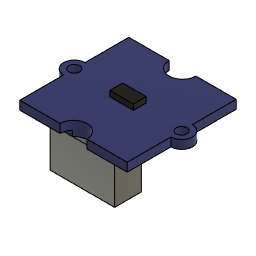
tofBreakoutBoard v3 (Autodesk Fusion 360 design; units mm, degrees)
Autodesk Fusion 360 part; units mm, degrees
sketch "Esquisse1" plane through (0, 0, 0) normal (0, 0, 1) x (1, 0, 0)
  line L0 (10, 13.25) -> (10, 7.05) construction
  line L1 (-3, 10.15) -> (23, 10.15) construction
  circle A0 centre (20, 10.15) radius 1
  circle A1 centre (0, 10.15) radius 1
  arc A2 (7.5, 20.3) -> (12.5, 20.3) centre (10, 20.3) ccw
  line L2 (20, 20.3) -> (12.5, 20.3)
  line L3 (7.5, 20.3) -> (0, 20.3)
  line L4 (20, 0) -> (20, 8.15)
  line L5 (20, 12.15) -> (20, 20.3)
  arc A3 (20, 8.15) -> (20, 12.15) centre (20, 10.15) ccw
  line L6 (0, 0) -> (7.5, 0)
  line L7 (12.5, 0) -> (20, 0)
  arc A4 (12.5, 0) -> (7.5, 0) centre (10, 0) ccw
  line L8 (0, 20.3) -> (0, 12.15)
  line L9 (0, 8.15) -> (0, 0)
  arc A5 (0, 12.15) -> (0, 8.15) centre (0, 10.15) ccw
  line L10 (0, 0) -> (20, 20.3) construction
  line L11 (0, 20.3) -> (20, 0) construction
  dimension "d1" = 20
  dimension "d2" = 20.3
  dimension "d3" = 5
  dimension "d4" = 5
  dimension "d5" = 4
  dimension "d6" = 4
  dimension "d7" = 2
  dimension "d8" = 2
  constraint horizontal L6
  constraint vertical L4
  constraint horizontal L2
  constraint vertical L8
  constraint coincident L6.start L9.end
  constraint parallel L0 L4
  constraint horizontal L1
  constraint concentric A0 A3
  constraint concentric A1 A5
  constraint coincident A2.start L2
  constraint collinear L2 L3
  constraint collinear L4 L5
  constraint coincident A0.centre L4
  constraint collinear L6 L7
  constraint coincident A4.centre L6
  constraint coincident A1.centre L8
  constraint midpoint L1 L10
  constraint midpoint L0 L1
  constraint coincident L0 A2.centre
  constraint coincident L0 A4.centre
  constraint coincident L1 A0.centre
  constraint coincident L1 A1.centre
  constraint collinear L8 L9
  constraint coincident A2.centre L2
  measures "d1" distance of L2.start L3.end
  measures "d2" distance of L4.start L2.start
  measures "d3" diameter of A4
  measures "d4" diameter of A2
  measures "d5" diameter of A3
  measures "d6" diameter of A5
  measures "d7" diameter of A1
  measures "d8" diameter of A0
extrude "Extrusion1" add sketch "Esquisse1" along normal blind 1.6 makes body 1
sketch "Esquisse2" plane through (0, 0, 1.6) normal (0, 0, 1) x (-1, 0, 0)
  circle A0 centre (-20, -10.15) radius 1
  circle A1 centre (0, -10.15) radius 1
  line L0 (-7.5, -20.3) -> (0, -20.3)
  line L1 (0, -20.3) -> (0, -12.15)
  arc A2 (0, -12.15) -> (0, -8.15) centre (0, -10.15) ccw
  line L2 (0, -8.15) -> (0, 0)
  line L3 (0, 0) -> (-7.5, 0)
  arc A3 (-12.5, 0) -> (-7.5, 0) centre (-10, 0) ccw
  line L4 (-12.5, 0) -> (-20, 0)
  line L5 (-20, 0) -> (-20, -8.15)
  arc A4 (-20, -8.15) -> (-20, -12.15) centre (-20, -10.15) ccw
  line L6 (-20, -12.15) -> (-20, -20.3)
  line L7 (-20, -20.3) -> (-12.5, -20.3)
  arc A5 (-7.5, -20.3) -> (-12.5, -20.3) centre (-10, -20.3) ccw
  line L8 (0, 0) -> (-20, -20.3) construction
  line L9 (0, -20.3) -> (-20, 0) construction
  line L10 (-12.2, -8.95) -> (-7.8, -8.95)
  line L11 (-7.8, -8.95) -> (-7.8, -11.35)
  line L12 (-7.8, -11.35) -> (-12.2, -11.35)
  line L13 (-12.2, -11.35) -> (-12.2, -8.95)
  line L14 (-12.2, -8.95) -> (-7.8, -11.35) construction
  line L15 (-7.8, -8.95) -> (-12.2, -11.35) construction
  point P0 (-10, -10.15)
  dimension "d11" = 4.4
  dimension "d12" = 2.4
  constraint coincident L2.end L3.start
  constraint coincident L6.end L7.start
  constraint coincident L0.end L1.start
  constraint coincident L4.end L5.start
  constraint horizontal L10
  constraint perpendicular L10 L11
  constraint parallel L10 L12
  constraint parallel L11 L13
  constraint coincident L14 P0
  constraint coincident L15 P0
  constraint midpoint L9 P0
  measures "d11" distance of L11.end L12.end
  measures "d12" distance of L10.start L12.end
extrude "Extrusion2" add sketch "Esquisse2" along normal blind 1 separate body contours L10 L11 L12 L13 makes body 2
sketch "Esquisse3" plane through (0, 0, 0) normal (0, 0, -1) x (1, 0, 0)
  circle A0 centre (20, -10.15) radius 1
  circle A1 centre (0, -10.15) radius 1
  line L0 (0, -20.3) -> (7.5, -20.3)
  arc A2 (12.5, -20.3) -> (7.5, -20.3) centre (10, -20.3) ccw
  line L1 (12.5, -20.3) -> (20, -20.3)
  line L2 (20, -20.3) -> (20, -12.15)
  arc A3 (20, -12.15) -> (20, -8.15) centre (20, -10.15) ccw
  line L3 (20, -8.15) -> (20, 0)
  line L4 (20, 0) -> (12.5, 0)
  arc A4 (7.5, 0) -> (12.5, 0) centre (10, 0) ccw
  line L5 (7.5, 0) -> (0, 0)
  line L6 (0, 0) -> (0, -8.15)
  arc A5 (0, -8.15) -> (0, -12.15) centre (0, -10.15) ccw
  line L7 (0, -12.15) -> (0, -20.3)
  line L8 (2.5, -1.65) -> (17.5, -1.65)
  line L9 (17.5, -1.65) -> (17.5, -18.65)
  line L10 (17.5, -18.65) -> (2.5, -18.65)
  line L11 (2.5, -18.65) -> (2.5, -1.65)
  line L12 (0, 0) -> (20, -20.3) construction
  line L13 (0, -20.3) -> (20, 0) construction
  line L14 (2.5, -1.65) -> (17.5, -18.65) construction
  line L15 (2.5, -18.65) -> (17.5, -1.65) construction
  dimension "d15" = 15
  dimension "d16" = 17
  constraint horizontal L8
  constraint vertical L9
  constraint horizontal L10
  constraint vertical L11
  constraint coincident L5.end L6.start
  constraint coincident L1.end L2.start
  constraint coincident L0.start L7.end
  constraint coincident L3.end L4.start
  constraint midpoint L12 L15
  measures "d15" distance of L8.start L8.end
  measures "d16" distance of L8.end L9.end
extrude "Extrusion3" add sketch "Esquisse3" along normal blind 1 contours A2 A4 L8 L9 L10 L11 bodies 1
sketch "Esquisse4" plane through (0, 0, -1) normal (0, 0, -1) x (1, 0, 0)
  line L0 (2.5, -18.65) -> (8.1218, -18.65)
  arc A0 (11.8782, -18.65) -> (8.1218, -18.65) centre (10, -20.3) ccw
  line L1 (11.8782, -18.65) -> (17.5, -18.65)
  line L2 (17.5, -18.65) -> (17.5, -1.65)
  line L3 (17.5, -1.65) -> (11.8782, -1.65)
  arc A1 (8.1218, -1.65) -> (11.8782, -1.65) centre (10, 0) ccw
  line L4 (8.1218, -1.65) -> (2.5, -1.65)
  line L5 (2.5, -1.65) -> (2.5, -18.65)
  line L6 (4, -6.65) -> (16, -6.65)
  line L7 (16, -6.65) -> (16, -1.65)
  line L8 (16, -1.65) -> (4, -1.65)
  line L9 (4, -1.65) -> (4, -6.65)
  line L10 (10, 6.5949) -> (10, -9.8949) construction
  dimension "d19" = 12
  dimension "d20" = 5
  constraint horizontal L6
  constraint vertical L7
  constraint horizontal L8
  constraint vertical L9
  constraint coincident L3 L7.end
  constraint coincident A1.centre L10
  constraint midpoint L8 L10
  constraint vertical L10
  measures "d19" distance of L6.start L6.end
  measures "d20" distance of L6.start L8.end
extrude "Extrusion4" add sketch "Esquisse4" along normal blind 7.5 separate body contours L3 A1 L4 L6 L7 L8 L9 | A1 L8 makes body 3
equation "d4 = d3"
